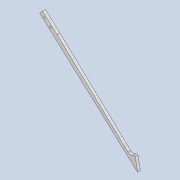
# Autodesk Inventor part: アーム先端
Saved by Autodesk Inventor 2020.4 (Build 244396000, 396)
## iProperties
Created: 2021-05-06
Part Number: アーム先端
Material: アルミニウム 7075
Document SubType Name: Modeling
Designer: happy
Density: 2.81 g/cm^3
Appearance: サテン - ブラシ仕上げ 重厚
Author: happy
Autodesk Inventor part; units mm, degrees
ref_plane "YZ Plane" through (0, 0, 0) normal (1, 0, 0) x (0, 1, 0)
ref_plane "XZ Plane" through (0, 0, 0) normal (0, 1, 0) x (-1, 0, 0)
ref_plane "XY Plane" through (0, 0, 0) normal (0, 0, 1) x (1, 0, 0)
sketch "スケッチ2" plane through (0, 0, 0) normal (0, 0, 1) x (1, 0, 0)
  line L0 (301.9981, -108.1255) -> (298.4342, -112.0532) construction
  line L1 (301.985, -108.1401) -> (343.1845, -145.5239)
  line L2 (185.1065, 0.6143) -> (481.3339, -268.178)
  line L3 (481.3339, -268.178) -> (468.2939, -282.5491)
  line L4 (333.6375, -147.6637) -> (289.2034, -107.3448)
  line L5 (333.6375, -147.6637) -> (474.6141, -275.5837)
  line L6 (301.985, -108.1401) -> (296.6091, -114.0646)
  line L7 (328.4554, -132.159) -> (477.974, -271.8809)
  line L8 (301.0696, -90.1631) -> (333.6375, -147.6637)
  line L9 (474.6141, -275.5837) -> (468.9509, -246.1231)
  arc A0 (457.2974, -252.559) -> (468.9509, -246.1231) centre (462.0767, -247.4445) ccw
  circle A1 centre (305.2216, -116.4782) radius 1.5
  circle A2 centre (316.3301, -126.5579) radius 1.5
  point P0 (0, 0)
  point P1 (0, 0)
  point P2 (321.0497, -125.4392)
  point P3 (299.297, -111.1023)
  point P4 (300.2162, -110.0894)
  dimension "d4" = 5
  dimension "d5" = 10
  dimension "d6" = 7
  dimension "d7" = 30
  constraints: 20 end point, 8 point on line, 3 centre point, 2 midpoint, 2 perpendicular, 2 point on circle, 2 tangent, 11 other
  measures "d4" distance of L5.end L7.end
  measures "d5" distance of L7.start point (321.05, -125.439)
  measures "d6" radius of A0
  measures "d7" distance of L5.end L9.end
extrude "押し出し1" add sketch "スケッチ2" along normal blind 5 contours L1 L8 L4 L6 | L1 L7 L9 L5 L8 | A0 L2 L9 L7 | A0 L9 L2
fillet "フィレット1" radius 2 1 edges at (468.9509, -246.1231, 2.5)
